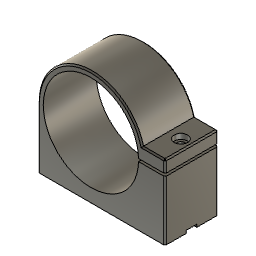
モーターマウント(外側) (Autodesk Fusion 360 design; units mm, degrees)
Autodesk Fusion 360 part; units mm, degrees
note: some values were not read from the file. Chosen so that the rebuilt part matches the saved one: which face or edge a step refers to. Set by a fixed rule: which sketch regions a step uses.
sketch "スケッチ1" plane through (0, 0, 0) normal (0, 1, 0) x (1, 0, 0)
  line L0 (0, 20) -> (0, 18)
  line L1 (20, -5) -> (28, -5)
  line L2 (20, -5) -> (19.3649, -5)
  line L3 (-20, 23) -> (0, 23)
  line L4 (0, 20) -> (0, 18)
  line L5 (28, 18) -> (28, 23)
  line L6 (28, 23) -> (0, 23)
  line L7 (0, 20) -> (0, 18)
  line L8 (-20, 0) -> (-20, 18)
  arc A0 (-20, 0) -> (19.3649, -5) centre (0, 0) ccw
  line L9 (-20, 18) -> (-20, 23)
  line L10 (28, -0.5) -> (17.9931, -0.5)
  line L11 (17.9931, 0.5) -> (28, 0.5)
  arc A1 (17.9931, 0.5) -> (17.9931, -0.5) centre (0, 0) ccw
  line L12 (28, -5) -> (28, -0.5)
  line L13 (28, 0.5) -> (28, 20)
  dimension "d1" = 36
  dimension "d4" = 5
  constraint coincident A0.centre A1.centre
  constraint vertical L0
  constraint perpendicular L1 L12
  constraint horizontal L3
  constraint vertical L4
  constraint coincident L0.end A1
  constraint vertical L5
  constraint horizontal L6
  constraint vertical L7
  constraint perpendicular L3 L9
  constraint coincident L11.end L12
  constraint perpendicular L11 L12
  constraint collinear L12 L13
  measures "d1" diameter of A1
  measures "d4" distance of L0.end L3.end
extrude "押し出し1" add sketch "スケッチ1" along normal blind 20
sketch "スケッチ2" plane through (0, 0, 5) normal (0, 0, 1) x (-1, 0, 0)
  line L0 (-19.3649, 0) -> (-28, 0)
  line L1 (-28, 0) -> (-28, -20)
  line L2 (-28, -20) -> (-19.3649, -20)
  line L3 (-19.3649, -20) -> (-19.3649, 0)
  circle A0 centre (-24, -10) radius 2.5
  dimension "d7" = 5
  measures "d7" diameter of A0
extrude "押し出し2" cut sketch "スケッチ2" against normal blind 2 contours A0
sketch "スケッチ3" plane through (0, 0, 3) normal (0, 0, 1) x (-1, 0, 0)
  circle A0 centre (-24, -10) radius 2.5
  circle A1 centre (-24, -10) radius 1.5
  dimension "d10" = 3
  constraint concentric A0 A1
  measures "d10" diameter of A1
extrude "押し出し3" cut sketch "スケッチ3" against normal blind 26 contours A1
sketch "スケッチ5" plane through (0, 0, 0) normal (0, 1, 0) x (1, 0, 0)
  line L0 (28, 23) -> (-20, 23)
  line L1 (-20, 23) -> (-20, 19)
  line L2 (-20, 19) -> (28, 19)
  line L3 (28, 19) -> (28, 23)
  constraint horizontal L0
  constraint vertical L1
  constraint horizontal L2
  constraint vertical L3
sketch "スケッチ8" plane through (0, 0, -23) normal (0, 0, -1) x (1, 0, 0)
  line L0 (0, -20) -> (0, 0)
  line L1 (-20, 0) -> (-20, -20)
  line L2 (28, -10) -> (24, -10)
  line L3 (26.8, -8.3834) -> (24, -6.7668)
  line L4 (24, -6.7668) -> (21.2, -8.3834)
  line L5 (21.2, -8.3834) -> (21.2, -11.6166)
  line L6 (21.2, -11.6166) -> (24, -13.2332)
  line L7 (24, -13.2332) -> (26.8, -11.6166)
  line L8 (26.8, -11.6166) -> (26.8, -8.3834)
  line L9 (0, 0) -> (-20, 0)
  line L10 (-20, -20) -> (0, -20)
  point P0 (24, -10)
  dimension "d20" = 4
  dimension "d21" = 2.8
  constraint coincident P0 L2.end
  measures "d20" distance of L2.start P0
  measures "d21" distance of P0 L8
extrude "押し出し6" cut sketch "スケッチ8" against normal blind 15 contours L3 L4 L5 L6 L7 L8
sketch "スケッチ9" plane through (0, 0, -19) normal (0, 0, 1) x (-1, 0, 0)
  line L0 (-28, 0) -> (20, 0)
  line L1 (20, 0) -> (20, 10)
  line L2 (20, 10) -> (-28, 10)
  line L3 (-28, 10) -> (-28, 0)
  line L4 (-35, -10) -> (25, -10)
  circle A0 centre (-23, 5) radius 1.5
  circle A1 centre (15, 5) radius 1.5
  circle A2 centre (-23, -25) radius 1.5
  circle A3 centre (15, -25) radius 1.5
  dimension "d24" = 3
  dimension "d25" = 3
  constraint horizontal L4
  constraint symmetric L4 A0 A2
  constraint symmetric L4 A1 A3
  measures "d24" diameter of A0
  measures "d25" diameter of A1
extrude "押し出し7" cut sketch "スケッチ9" against normal blind 4 contours A0 | A1 | A2 | A3
chamfer "面取り1" distance 0.5 angle 45 11 edges at (23.6825, 0, 5) (28, 10, 5) (23.6825, 20, 5) (-2.5201, 0, 19.8406) (-2.5201, 20, 19.8406) (28, 0, 2.75) (28, 0, -11.75) (-20, 0, -11.5) (28, 20, 2.75) (28, 20, -11.75) (-20, 20, -11.5)
sketch "スケッチ10" plane through (0, 0, -23) normal (0, 0, -1) x (1, 0, 0)
  line L0 (-19.5, 0) -> (-20, -0.5)
  line L1 (-20, -0.5) -> (-20, -19.5)
  line L2 (-20, -19.5) -> (-19.5, -20)
  line L3 (-19.5, -20) -> (0, -20)
  line L4 (0, -20) -> (0, 0)
  line L5 (0, 0) -> (-19.5, 0)
  line L6 (-19.5, -20) -> (-20, -20)
  line L7 (28, -17) -> (28, -20)
  line L8 (-20, -20) -> (-15, -20)
  line L9 (-20, 0) -> (-20, -3)
  line L10 (28, -20) -> (28, -17)
  line L11 (-20, -20) -> (-20, -19.5)
  line L12 (-20, -0.5) -> (-20, 0)
  line L13 (-20, 0) -> (-19.5, 0)
  circle A0 centre (23, -17) radius 1
  circle A1 centre (-15, -17) radius 1
  circle A2 centre (23, -3) radius 1
  circle A3 centre (-15, -3) radius 1
  dimension "d34" = 5
  dimension "d41" = 2
  dimension "d42" = 2
  dimension "d43" = 2
  dimension "d44" = 2
  constraint horizontal L6
  constraint vertical L11
  constraint horizontal L13
  constraint vertical L7
  constraint coincident L3 L8.end
  constraint coincident L1 L9.end
  constraint coincident L9.end L11
  constraint collinear L11 L12
  measures "d34" distance of L7.start A0.centre
  measures "d41" diameter of A0
  measures "d42" diameter of A1
  measures "d43" diameter of A2
  measures "d44" diameter of A3
extrude "押し出し10" cut sketch "スケッチ10" against normal blind 10 contours A0 | A1 | A2 | A3
sketch "スケッチ12" plane through (0, 0, -23) normal (0, 0, -1) x (1, 0, 0)
  circle A0 centre (-15, -17) radius 1
  circle A1 centre (-15, -3) radius 1
  line L0 (-19.5, 0) -> (-20, -0.5)
  line L1 (-20, -0.5) -> (-20, -19.5)
  line L2 (-20, -19.5) -> (-19.5, -20)
  line L3 (-19.5, -20) -> (0, -20)
  line L4 (0, -20) -> (0, 0)
  line L5 (0, 0) -> (-19.5, 0)
  line L6 (-20, -12) -> (28, -12)
  line L7 (28, -12) -> (28, -8)
  line L8 (28, -8) -> (-20, -8)
  line L9 (-20, -8) -> (-20, -12)
  dimension "d47" = 48
  dimension "d48" = 4
  constraint horizontal L6
  constraint vertical L7
  constraint horizontal L8
  constraint vertical L9
  constraint coincident L1 L6.start
  measures "d47" distance of L6.start L6.end
  measures "d48" distance of L6.start L8.end
extrude "押し出し11" cut sketch "スケッチ12" against normal blind 1 contours L1 L4 L6 L8 L9 | L4 L6 L7 L8
